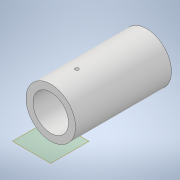
# Autodesk Inventor part: threaf-f
Saved by Autodesk Inventor 2022 (Build 260153000, 153)
## iProperties
Created: 2021-10-07
Part Number: threaf-f
Material: Generic
Document SubType Name: Modeling
Designer: tecware
Density: 1 g/cm^3
Appearance: Default
Author: tecware
## iProperties of the stored document threaf-f_3DPrint.ipt
Created: 2021-10-07
Part Number: threaf-f_3DPrint
Material: Generic
Document SubType Name: Modeling
Designer: tecware
Density: 1 g/cm^3
Appearance: Default
Author: tecware
Autodesk Inventor part; units mm, degrees
ref_plane "YZ Plane" through (0, 0, 0) normal (1, 0, 0) x (0, 1, 0)
ref_plane "XZ Plane" through (0, 0, 0) normal (0, 1, 0) x (-1, 0, 0)
ref_plane "XY Plane" through (0, 0, 0) normal (0, 0, 1) x (1, 0, 0)
sketch "Sketch1" plane through (0, 0, 0) normal (0, 0, 1) x (1, 0, 0)
  circle A0 centre (0, 0) radius 11
  circle A1 centre (0, 0) radius 14.2
  dimension "d23" = 22
  dimension "d81" = 28.4
  constraints: 2 centre point, 2 coincident
  measures "d23" diameter of A0
  measures "d81" diameter of A1
extrude "Bottom" add sketch "Sketch1" along normal blind 10
thread "Thread4" size "M22x3" class "6H" standard "ANSI Metric M Profile" full length
sketch "Sketch13" plane through (0, 0, 10) normal (-1, 0, 0) x (0, 1, 0)
  line L0 (11, 0) -> (11, 10)
  line L1 (11, 10) -> (8.7756, 10)
  line L2 (8.7756, 10) -> (8.7756, 0)
  line L3 (8.7756, 0) -> (11, 0)
  line L4 (0, -2) -> (0, 12) projected
  constraints: 8 end point
revolve "Revolution6" add sketch "Sketch13" angle 360 about axis through (0, 0, 10) along (0, 0, -1) separate body
sketch "Sketch12" plane through (0, 11, 10) normal (1, 0, 0) x (0, 0, -1)
  line L0 (-1.7501, -0.1519) -> (-1.5001, -0.1519) construction
  line L1 (0.2499, -2.0728) -> (-0.0001, -2.5531) construction
  line L2 (-3.0001, -2.5531) -> (-3.2501, -2.0728) construction
  line L3 (-1.2501, -0.1519) -> (-1.5001, 0.3284) construction
  line L4 (-1.5001, 0.3284) -> (-1.7501, -0.1519) construction
  line L5 (-3.0001, -2.5531) -> (-2.7501, -2.0728) construction
  line L6 (-1.2501, -0.1519) -> (-0.2501, -2.0728)
  line L7 (-3.2501, -2.0728) -> (-2.7501, -2.0728) construction
  arc A0 (-3.2501, -2.0728) -> (-3.0001, -2.2246) centre (-3.0001, -1.9427) ccw construction
  line L8 (0.2499, -2.0728) -> (-0.2501, -2.0728) construction
  line L9 (-3.0001, -2.5531) -> (-3.0001, -2.0728) construction
  line L10 (-0.0001, -2.5531) -> (-0.0001, -2.0728) construction
  line L11 (-1.5001, 0.3284) -> (-1.5001, -0.0002) construction
  line L12 (-3.0001, -2.2246) -> (-0.0001, -2.2246)
  arc A1 (-3.0001, -2.2246) -> (-2.7501, -2.0728) centre (-3.0001, -1.9427) ccw
  line L13 (-0.2501, -2.0728) -> (-0.0001, -2.5531) construction
  line L14 (-2.7501, -2.0728) -> (-1.7501, -0.1519)
  line L15 (-0.0001, -0.0002) -> (-0.0001, 0.0177)
  line L16 (-0.0001, 0.0177) -> (-0.0001, -0.0002)
  line L17 (-0.0001, -0.0002) -> (0.0334, -0.0002)
  arc A2 (-0.2501, -2.0728) -> (-0.0001, -2.2246) centre (-0.0001, -1.9427) ccw
  arc A3 (-0.0001, -2.2246) -> (0.2499, -2.0728) centre (-0.0001, -1.9427) ccw construction
  arc A4 (-1.5001, -0.0002) -> (-1.7501, -0.1519) centre (-1.5001, -0.282) ccw
  arc A5 (-1.2501, -0.1519) -> (-1.5001, -0.0002) centre (-1.5001, -0.282) ccw
  line L18 (-1.5001, -0.0002) -> (-1.5001, -0.1519) construction
  line L19 (-1.5001, -0.1519) -> (-1.2501, -0.1519) construction
  dimension "d104" = 55
  dimension "d105" = 0.4803
  dimension "d106" = 0.4803
  dimension "Sketch12_ThreadOffset" = 0
  dimension "Sketch12_MajorRadius" = 2.2244
  dimension "d109" = 3
  dimension "Sketch12_MinorRadius" = 0
  constraints: 40 end point, 12 point on circle, 10 parallel, 8 tangent, 6 centre point, 6 collinear, 2 midpoint, 2 point on line, 1 horizontal, 1 perpendicular, 3 other
  measures "d104" angle of L6 L14
  measures "d105" distance of L3.end L0.end
  measures "d106" distance of L1.end L10.end
  measures "Sketch12_ThreadOffset" distance between parallel lines of L15 L10
  measures "Sketch12_MajorRadius" distance from line of L12 L15.start
  measures "d109" distance from line of L1.end L9
  measures "Sketch12_MinorRadius" distance edge to line of A5 L17
coil "Coil6" sketch "Sketch12" operation cut axis through (0, 0, 10) along (0, 0, -1) pitch 3.003 turns 5.328005 hand right bodies 2
sketch "Sketch14" plane through (0, 0, 10) normal (0, 0, 1) x (1, 0, 0)
  circle A0 centre (0, 0) radius 11
  circle A1 centre (0, 0) radius 14.2
  dimension "d130" = 22
  dimension "d131" = 28.4
  constraints: 2 centre point, 2 coincident
  measures "d130" diameter of A0
  measures "d131" diameter of A1
extrude "Mid" add sketch "Sketch14" along normal blind 20 bodies 1
sketch "Sketch15" plane through (0, 0, 30) normal (0, 0, 1) x (1, 0, 0)
  circle A0 centre (0, 0) radius 10.2
  circle A1 centre (0, 0) radius 14.2
  dimension "d124" = 20.4
  dimension "d125" = 28.4
  constraints: 2 centre point, 2 coincident
  measures "d124" diameter of A0
  measures "d125" diameter of A1
extrude "Top" add sketch "Sketch15" along normal blind 30 bodies 1
sketch "Sketch16" plane through (0, 0, 30) normal (0, 0, 1) x (1, 0, 0)
  circle A0 centre (0, 0) radius 11
  circle A1 centre (0, 0) radius 9
  dimension "d133" = 22
  dimension "d134" = 18
  constraints: 2 centre point, 2 coincident
  measures "d133" diameter of A0
  measures "d134" diameter of A1
extrude "Extrusion4" add sketch "Sketch16" along normal blind 2 bodies 1
fillet "Fillet4" radius 5 2 edges at (-11, 0, 30) (-9, 0, 30)
ref_plane "Work Plane1" through (0, -14.2, 55) normal (0, -1, 0) x (1, 0, 0)
sketch "Sketch18" plane through (0, -14.2, 55) normal (0, -1, 0) x (1, 0, 0)
  line L0 (14.2, 5) -> (-14.2, 5) projected
  point P0 (0, -55)
  point P1 (0, -10)
  dimension "d138" = 15
  measures "d138" distance from line of L0 point (0, -10)
hole "Hole1" at (0, -14.2, 45) direction (0, 1, 0) diameter 2 end through all bodies 1
equation "\"d104\" = d111"
equation "\"d105\" = 0.160083 * Sketch12_Pitch"
equation "\"d106\" = 0.160083 * Sketch12_Pitch"
equation "\"d109\" = Sketch12_Pitch"
equation "\"d12\" = 55deg"
equation "\"Sketch2_Pitch\" = 1.5"
equation "\"d31\" = 55deg"
equation "\"Sketch4_Pitch\" = 1.5"
equation "\"d52\" = 55deg"
equation "\"Sketch6_Pitch\" = 2.5"
equation "\"d70\" = 55deg"
equation "\"Sketch8_Pitch\" = 2.5"
equation "\"d91\" = 55deg"
equation "\"Sketch10_Pitch\" = 3"
equation "\"d111\" = 55deg"
equation "\"Sketch12_Pitch\" = 3"
body "Solid1"
body "Solid7"
